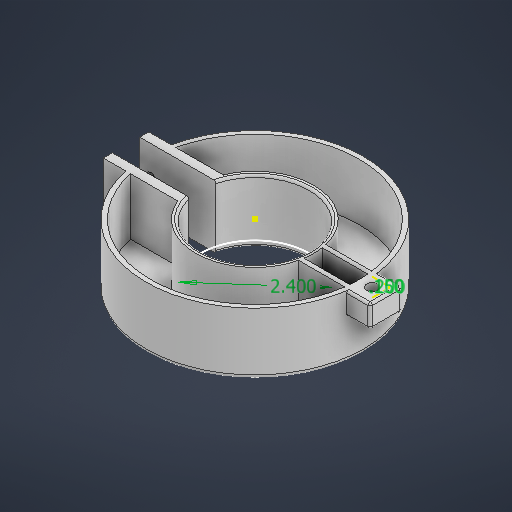
# Autodesk Inventor part: Bouy versioun 14
Saved by Autodesk Inventor 2026 (Build 300175050, 175E)
## iProperties
Created: 2025-06-16
Part Number: Bouy versioun 14
Material: Generic
Document SubType Name: Modeling
Designer: localuser
Density: 1 g/cm^3
Appearance: Default
Author: localuser
Autodesk Inventor part; units mm, degrees
ref_plane "YZ Plane" through (0, 0, 0) normal (1, 0, 0) x (0, 1, 0)
ref_plane "XZ Plane" through (0, 0, 0) normal (0, 1, 0) x (-1, 0, 0)
ref_plane "XY Plane" through (0, 0, 0) normal (0, 0, 1) x (1, 0, 0)
sketch "Sketch2" plane through (0, 0, 0) normal (0, 1, 0) x (-1, 0, 0)
  circle A0 centre (0, 0) radius 30.48
  dimension "d4" = 60.96
  constraints: 1 centre point, 1 coincident
  measures "d4" diameter of A0
sketch "Sketch3" plane through (0, 0, 0) normal (0, 1, 0) x (-1, 0, 0)
  line L0 (0, 0) -> (30.48, 0)
  line L1 (30.48, 0) -> (30.48, 12.7)
  line L2 (30.48, 12.7) -> (30.48, -12.7)
  line L3 (30.48, -12.7) -> (27.3484, -12.7)
  line L4 (27.3484, -12.7) -> (30.48, -12.7)
  line L5 (30.48, 12.7) -> (27.3484, 12.7)
  line L6 (27.3484, 12.7) -> (27.3484, -12.7)
  circle A0 centre (0, 0) radius 33.02
  circle A1 centre (0, 0) radius 58.42
  circle A2 centre (0, 0) radius 60.96
  circle A3 centre (0, 0) radius 30.48
  line L7 (27.7081, 12.7) -> (30.48, 12.7)
  line L8 (30.48, -12.7) -> (27.7081, -12.7)
  arc A4 (27.7081, -12.7) -> (27.7081, 12.7) centre (0, 0) ccw
  line L9 (27.7081, -12.7) -> (72.1581, -12.7)
  line L10 (72.1581, -12.7) -> (72.1581, -7.62)
  line L11 (72.1581, -7.62) -> (30.48, -7.62)
  line L12 (27.7081, 12.7) -> (72.1581, 12.7)
  line L13 (72.1581, 12.7) -> (72.1581, 7.62)
  line L14 (72.1581, 7.62) -> (30.48, 7.62)
  circle A5 centre (0, 0) radius 58.42
  circle A6 centre (0, 0) radius 60.96
  line L15 (60.4819, -7.62) -> (57.9209, -7.62)
  line L16 (59.6224, -12.7) -> (57.0229, -12.7)
  line L17 (59.6224, 12.7) -> (57.0229, 12.7)
  line L18 (60.4819, 7.62) -> (57.9209, 7.62)
  line L19 (32.1287, 7.62) -> (29.5121, 7.62)
  line L20 (30.48, -7.62) -> (29.5121, -7.62)
  point P0 (59.6224, 12.7)
  point P1 (59.6224, -12.7)
  point P2 (57.0229, -12.7)
  point P3 (57.0229, 12.7)
  dimension "d6" = 30.48
  dimension "d7" = 12.7
  dimension "d8" = 25.4
  dimension "d9" = 66.04
  dimension "d10" = 116.84
  dimension "d11" = 121.92
  dimension "d12" = 60.96
  dimension "d13" = 44.45
  dimension "d14" = 5.08
  dimension "d15" = 44.45
  dimension "d16" = 5.08
  constraints: 42 end point, 18 point on circle, 18 point on line, 7 centre point, 7 coincident, 7 perpendicular, 2 concentric, 2 horizontal, 2 parallel, 1 collinear
  measures "d6" distance of L0.start L0.end
  measures "d7" distance of L0.end L1.end
  measures "d8" distance of L1.end L2.end
  measures "d9" diameter of A0
  measures "d10" diameter of A1
  measures "d11" diameter of A2
  measures "d12" diameter of A3
  measures "d13" distance of L9.start L9.end
  measures "d14" distance of L9.end L10.end
  measures "d15" distance of L7.start L12.end
  measures "d16" distance of L12.end L13.end
extrude "Extrusion1" add sketch "Sketch3" along normal blind 31.75 contours L19 A3 L5 L1 | L1 A0 L14 | L11 A0 L2 | L2 L3 A3 L20 | A3 L3 A0 L5 | L12 A1 L14 A0 | A0 L11 A1 L9 | L12 A2 L14 A1 | A1 L9 A2 L12 | A1 L11 A2 L9 | L12 L13 L14 A2 | A2 L11 L10 L9
sketch "Sketch4" plane through (0, 31.75, 0) normal (0, 1, 0) x (1, 0, 0)
  arc A0 (-29.5121, -7.62) -> (-29.5121, 7.62) centre (0, 0) ccw projected
  line L0 (-29.5121, 7.62) -> (60.4819, 7.62)
  arc A1 (-59.6224, -12.7) -> (-59.6224, 12.7) centre (0, 0) ccw projected
  line L1 (-29.5121, 7.62) -> (-29.5121, 10.16)
  line L2 (-29.5121, 10.16) -> (60.4819, 10.16)
  line L3 (60.4819, 10.16) -> (60.4819, 7.62)
  arc A2 (-57.0229, -12.7) -> (-57.0229, 12.7) centre (0, 0) ccw projected
  circle A3 centre (0, 0) radius 58.42
  arc A4 (57.9209, 7.62) -> (57.5297, 10.16) centre (0, 0) ccw
  circle A5 centre (0, 0) radius 33.02
  arc A6 (-30.48, -12.7) -> (-30.48, 12.7) centre (0, 0) ccw projected
  arc A7 (32.1287, 7.62) -> (31.4181, 10.16) centre (0, 0) ccw
  line L4 (-29.5121, -7.62) -> (57.9209, -7.62)
  line L5 (57.9209, -7.62) -> (57.5349, -10.1305)
  line L6 (57.9209, -7.62) -> (57.9209, -10.16)
  line L7 (57.9209, -10.16) -> (-28.7368, -10.16)
  arc A8 (-29.5121, -7.62) -> (-29.5121, 7.62) centre (0, 0) ccw projected
  arc A9 (31.4181, -10.16) -> (32.1287, -7.62) centre (0, 0) ccw
  arc A10 (57.5349, -10.1305) -> (57.9209, -7.62) centre (0, 0) ccw
  point P0 (32.1287, -7.62)
  point P1 (57.9209, 7.62)
  point P2 (32.1287, 7.62)
  dimension "d19" = 2.54
  dimension "d20" = 2.54
  dimension "d21" = 2.54
  constraints: 18 point on circle, 16 end point, 6 centre point, 6 point on line, 4 perpendicular, 2 coincident, 2 horizontal, 1 concentric, 1 vertical
  measures "d19" distance of L0.start L1.end
  measures "d20" distance of L4.end L5.end
  measures "d21" distance of L4.end L6.end
extrude "Extrusion2" add sketch "Sketch4" against normal blind 31.75 contours A5 L0 A2 L4
shell "Shell1" thickness 2.54 removed faces 1 at (48.7739, 31.75, 0)
sketch "Sketch5" plane through (0, 0, 0) normal (0, -1, 0) x (1, 0, 0)
  circle A0 centre (0, 0) radius 60.96
  arc A1 (-59.6224, -12.7) -> (-59.6224, 12.7) centre (0, 0) ccw projected
  circle A2 centre (0, 0) radius 30.48
  line L0 (-29.5121, 7.62) -> (-72.1581, 7.62) projected
  line L1 (-29.5121, 7.62) -> (-60.4819, 7.62)
  line L2 (-72.1581, -7.62) -> (-29.5121, -7.62) projected
  line L3 (-29.5121, -7.62) -> (-60.4819, -7.62)
  constraints: 4 end point, 2 centre point, 2 coincident, 2 point on circle, 2 point on line
extrude "Extrusion3" add sketch "Sketch5" along normal blind 3.175 contours A0 L2 A2 L0 picked at (40.9581, -29.698)
fillet "Fillet1" radius 2.54 1 edges at (60.96, -3.175, 0)
fillet "Fillet2" radius 1.27 1 edges at (30.48, -3.175, 0)
fillet "Fillet3" radius 1.27 1 edges at (30.48, 31.75, 0)
sketch "Sketch6" plane through (-59.6224, 0, -12.7) normal (0, 0, -1) x (-1, 0, 0)
  line L0 (12.5357, 0) -> (12.5357, 31.75) projected
  line L1 (12.5357, 31.75) -> (6.1857, 31.75)
  line L2 (0, 31.75) -> (12.5357, 31.75) projected
  line L3 (6.1857, 31.75) -> (6.1857, 15.24)
  point P0 (-59.6224, 0)
  dimension "d30" = 6.35
  dimension "d31" = 16.51
  constraints: 4 end point, 1 perpendicular, 1 point on line
  measures "d30" distance of L0.end L1.end
  measures "d31" distance of L1.end L3.end
hole "Hole1" at (-65.8081, 15.24, -12.7) direction (0, 0, 1) diameter 5.1054 end through all
sketch "Sketch7" plane through (0, 31.75, 0) normal (0, 1, 0) x (1, 0, 0)
  arc A0 (58.1987, -5.08) -> (58.1987, 5.08) centre (0, 0) ccw projected
  line L0 (58.1987, 5.08) -> (58.1987, -5.08)
  line L1 (58.1987, -5.08) -> (68.3587, -5.08)
  line L2 (68.3587, -5.08) -> (68.3587, 5.08)
  line L3 (68.3587, 5.08) -> (58.1987, 5.08)
  circle A1 centre (0, 0) radius 60.96
  arc A2 (60.748, -5.08) -> (60.748, 5.08) centre (0, 0) ccw
  dimension "d39" = 10.16
  constraints: 8 end point, 5 point on circle, 2 centre point, 2 perpendicular, 2 point on line, 1 coincident, 1 horizontal, 1 vertical
  measures "d39" distance of L0.end L1.end
extrude "Extrusion4" add sketch "Sketch7" against normal blind 12.7 contours A1 L3 L2 L1
sketch "Sketch9" plane through (68.3587, 31.75, 5.08) normal (1, 0, 0) x (0, 0, -1)
  line L0 (10.16, -29.21) -> (10.16, 0) projected
  line L1 (0, -12.7) -> (10.16, -12.7) projected
  line L2 (10.16, 0) -> (10.16, -12.7)
  line L3 (10.16, -12.7) -> (0, -12.7)
  line L4 (0, -12.7) -> (0, 0)
  line L5 (0, 0) -> (10.16, 0)
  point P0 (5.08, -31.75)
  dimension "d51" = 10.16
  dimension "d52" = 12.7
  constraints: 8 end point, 3 perpendicular
  measures "d51" distance of L1.end L3.end
  measures "d52" distance of L3.end L4.end
extrude "Extrusion5" add sketch "Sketch9" along normal blind 2.54
sketch "Sketch10" plane through (0, 31.75, 0) normal (0, 1, 0) x (1, 0, 0)
  line L0 (70.8987, -5.08) -> (70.8987, 5.08) projected
  line L1 (70.8987, 5.08) -> (67.0887, 5.08)
  line L2 (60.748, 5.08) -> (70.8987, 5.08) projected
  line L3 (67.0887, 5.08) -> (72.1687, 5.08)
  point P0 (0, 0)
  dimension "d55" = 3.81
  dimension "d56" = 5.08
  constraints: 4 end point, 2 point on line
  measures "d55" distance of L0.end L1.end
  measures "d56" distance of L1.end L3.end
sketch "Sketch11" plane through (0, 31.75, 0) normal (0, 1, 0) x (1, 0, 0)
  line L0 (60.748, -5.08) -> (70.8987, -5.08) projected
  line L1 (70.8987, -5.08) -> (65.8187, -5.08)
  line L2 (65.8187, -5.08) -> (65.8187, 0)
  point P0 (0, 0)
  dimension "d57" = 5.08
  dimension "d58" = 5.08
  constraints: 4 end point, 1 perpendicular, 1 point on line
  measures "d57" distance of L0.end L1.end
  measures "d58" distance of L1.end L2.end
hole "Hole3" at (65.8187, 31.75, 0) direction (0, -1, 0) diameter 6.35 end through all
sketch "Sketch12" plane through (0, 31.75, 0) normal (0, 1, 0) x (1, 0, 0)
  circle A0 centre (0, 0) radius 60.96
  line L0 (60.748, -5.08) -> (70.8987, -5.08) projected
  line L1 (70.8987, -5.08) -> (70.8987, -8.89)
  line L2 (70.8987, -8.89) -> (60.3083, -8.89)
  line L3 (70.8987, 5.08) -> (60.748, 5.08) projected
  line L4 (70.8987, 5.08) -> (70.8987, 7.1567)
  line L5 (70.8987, 5.08) -> (70.8987, 8.89)
  line L6 (70.8987, 8.89) -> (60.3083, 8.89)
  line L7 (70.8987, -8.89) -> (73.4387, -8.89)
  line L8 (73.4387, -8.89) -> (73.4387, 8.89)
  line L9 (73.4387, 8.89) -> (70.8987, 8.89)
  line L10 (70.8987, 5.08) -> (70.8987, -5.08) projected
  line L11 (70.8987, 5.08) -> (70.8987, -5.08)
  dimension "d66" = 3.81
  dimension "d67" = 3.81
  dimension "d68" = 2.54
  constraints: 18 end point, 4 perpendicular, 3 point on line, 2 point on circle, 1 centre point, 1 coincident, 1 collinear, 1 parallel, 1 vertical
  measures "d66" distance of L0.end L1.end
  measures "d67" distance of L3.start L5.end
  measures "d68" distance of L1.end L7.end
extrude "Extrusion6" add sketch "Sketch12" against normal blind 12.7 contours A0 L6 L5 L4 L3 | L0 L1 L2 A0 | L4 L5 L9 L8 L7 L1 L10
fillet "Fillet4" radius 1.27 8 edges at (66.8735, 31.75, 8.89) (73.4387, 31.75, 0) (66.8735, 31.75, -8.89) (73.4387, 25.4, 8.89) (66.8735, 19.05, 8.89) (73.4387, 19.05, 0) (66.8735, 19.05, -8.89) (73.4387, 25.4, -8.89)
body "Solid1"
